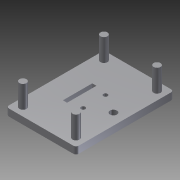
# Autodesk Inventor part: Platte
Saved by Autodesk Inventor 2011 (Build 150239000, 239)
## iProperties
Created: 2015-07-17
Part Number: Platte
Document SubType Name: Modeling
Designer: schmieder
Density: 1 g/cm^3
Author: schmieder
Autodesk Inventor part; units mm, degrees
ref_plane "YZ Plane" through (0, 0, 0) normal (1, 0, 0) x (0, 1, 0)
ref_plane "XZ Plane" through (0, 0, 0) normal (0, 1, 0) x (-1, 0, 0)
ref_plane "XY Plane" through (0, 0, 0) normal (0, 0, 1) x (1, 0, 0)
sketch "Skizze1" plane through (0, 0, 0) normal (0, 0, 1) x (1, 0, 0)
  line L0 (-20.1198, 0) -> (29.8802, 0)
  line L1 (29.8802, 0) -> (29.8802, 70)
  line L2 (29.8802, 70) -> (-20.1198, 70)
  line L3 (-20.1198, 70) -> (-20.1198, 0)
  point P0 (0, 0)
  dimension "d0" = 50
  dimension "d1" = 70
  constraints: 8 end point, 2 parallel, 1 horizontal, 1 perpendicular
  measures "d0" distance of L2.end L1.end
  measures "d1" distance of L1.end L0.end
extrude "Extrusion1" add sketch "Skizze1" along normal blind 5
fillet "Rundung1" radius 2 4 edges at (-20.1198, 0, 2.5) (29.8802, 0, 2.5) (29.8802, 70, 2.5) (-20.1198, 70, 2.5)
sketch "Skizze2" plane through (0, 0, 5) normal (0, 0, 1) x (1, 0, 0)
  line L0 (-3.9308, 24.4243) -> (-0.9308, 24.4243)
  line L1 (-0.9308, 24.4243) -> (-0.9308, 45.4243)
  line L2 (-0.9308, 45.4243) -> (-3.9308, 45.4243)
  line L3 (-3.9308, 45.4243) -> (-3.9308, 24.4243)
  point P0 (0, 0)
  dimension "d5" = 3
  dimension "d6" = 21
  constraints: 8 end point, 2 parallel, 1 horizontal, 1 perpendicular
  measures "d5" distance of L2.end L1.end
  measures "d6" distance of L1.end L0.end
extrude "Extrusion2" cut sketch "Skizze2" against normal up to surface (5 mm away)
sketch "Skizze3" plane through (0, 0, 5) normal (0, 0, 1) x (1, 0, 0)
  line L0 (-20.1198, 2) -> (-20.1198, 68) projected
  line L1 (27.8802, 0) -> (-18.1198, 0) projected
  line L2 (29.8802, 68) -> (29.8802, 2) projected
  line L3 (-18.1198, 70) -> (27.8802, 70) projected
  line L4 (-3.9308, 45.4243) -> (10.5692, 45.4243)
  line L5 (10.5692, 45.4243) -> (10.5692, 24.4243)
  line L6 (10.5692, 24.4243) -> (-3.9308, 24.4243)
  line L7 (-3.9308, 24.4243) -> (-3.9308, 45.4243)
  circle A0 centre (8.0692, 42.9243) radius 1.5
  circle A1 centre (8.0692, 26.9243) radius 1.5
  circle A2 centre (21.7604, 34.9243) radius 2.5
  circle A3 centre (-14.1198, 64) radius 2.5
  circle A4 centre (23.8802, 64) radius 2.5
  circle A5 centre (-14.1198, 6) radius 2.5
  circle A6 centre (23.8802, 6) radius 2.5
  point P0 (0, 0)
  dimension "d9" = 14.5
  dimension "d10" = 21
  dimension "d11" = 3
  dimension "d12" = 3
  dimension "d13" = 2.5
  dimension "d14" = 2.5
  dimension "d15" = 2.5
  dimension "d16" = 2.5
  dimension "d17" = 5
  dimension "d18" = 5
  dimension "d19" = 5
  dimension "d20" = 5
  dimension "d21" = 5
  dimension "d22" = 6
  dimension "d23" = 6
  dimension "d24" = 6
  dimension "d25" = 6
  dimension "d26" = 6
  dimension "d27" = 6
  dimension "d28" = 6
  dimension "d29" = 6
  constraints: 8 end point, 7 centre point, 2 parallel, 1 horizontal, 1 perpendicular
  measures "d9" distance of L5.end L6.end
  measures "d10" distance of L4.end L5.end
  measures "d11" diameter of A0
  measures "d12" diameter of A1
  measures "d13" distance from line of L4 A0.centre
  measures "d14" distance from line of L5 A0.centre
  measures "d15" distance from line of L5 A1.centre
  measures "d16" distance from line of L6 A1.centre
  measures "d17" diameter of A2
  measures "d18" diameter of A3
  measures "d19" diameter of A4
  measures "d20" diameter of A5
  measures "d21" diameter of A6
  measures "d22" distance from line of L3 A3.centre
  measures "d23" distance from line of L0 A3.centre
  measures "d24" distance from line of L2 A4.centre
  measures "d25" distance from line of L3 A4.centre
  measures "d26" distance from line of L2 A6.centre
  measures "d27" distance from line of L1 A6.centre
  measures "d28" distance from line of L0 A5.centre
  measures "d29" distance from line of L1 A5.centre
sketch "Skizze4" plane through (0, 0, 5) normal (0, 0, 1) x (1, 0, 0)
  circle A0 centre (-14.1198, 64) radius 2.5
  circle A1 centre (23.8802, 64) radius 2.5
  circle A2 centre (-14.1198, 6) radius 2.5
  circle A3 centre (23.8802, 6) radius 2.5
  point P0 (0, 0)
  dimension "d30" = 5
  dimension "d31" = 5
  dimension "d32" = 5
  dimension "d33" = 5
  constraints: 4 centre point
  measures "d30" diameter of A0
  measures "d31" diameter of A1
  measures "d32" diameter of A2
  measures "d33" diameter of A3
extrude "Extrusion3" add sketch "Skizze4" along normal blind 16
extrude "Extrusion4" cut sketch "Skizze3" against normal up to surface (5 mm away) contours A0 | A1 | A2
